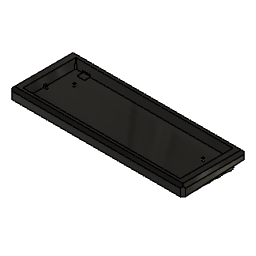
Guide_Poker (Autodesk Fusion 360 design; units mm, degrees)
Autodesk Fusion 360 part; units mm, degrees
sketch "スケッチ1" plane through (0, 0, 0) normal (0, 0, 1) x (1, 0, 0)
  line L0 (0, 0) -> (286.75, 0)
  line L1 (286.75, 0) -> (286.75, -96.25)
  line L2 (286.75, -96.25) -> (0, -96.25)
  line L3 (0, -96.25) -> (0, 0)
  line L4 (-15, 10) -> (301.75, 10)
  line L5 (301.75, 10) -> (301.75, -106.25)
  line L6 (301.75, -106.25) -> (-15, -106.25)
  line L7 (-15, -106.25) -> (-15, 10)
  circle A0 centre (260.95, -28.5) radius 2
  circle A1 centre (282.75, -57.25) radius 2
  circle A2 centre (191.45, -85.85) radius 2
  circle A3 centre (4, -57.25) radius 2
  circle A4 centre (26, -28.5) radius 2
  line L8 (286.75, -59.25) -> (282.75, -59.25)
  line L9 (286.75, -55.25) -> (282.75, -55.25)
  line L10 (0, -59.25) -> (4, -59.25)
  line L11 (0, -55.25) -> (4, -55.25)
  circle A5 centre (129, -47.75) radius 2
  circle A6 centre (4, -57.25) radius 0.9
  circle A7 centre (26, -28.5) radius 0.9
  circle A8 centre (191.45, -85.85) radius 0.9
  circle A9 centre (129, -47.75) radius 0.9
  circle A10 centre (282.75, -57.25) radius 0.9
  circle A11 centre (260.95, -28.5) radius 0.9
  dimension "d7" = 286.75
  dimension "d8" = 96.25
  dimension "d9" = 15
  dimension "d10" = 10
  dimension "d11" = 10
  dimension "d12" = 15
  dimension "d13" = 4
  dimension "d14" = 28.5
  dimension "d15" = 25.8
  dimension "d16" = 4
  dimension "d17" = 4
  dimension "d18" = 4
  dimension "d19" = 4
  dimension "d20" = 28.5
  dimension "d21" = 26
  dimension "d22" = 39
  dimension "d23" = 4
  dimension "d24" = 4
  dimension "d25" = 39
  dimension "d26" = 10.4
  dimension "d27" = 95.3
  dimension "d28" = 4
  dimension "d29" = 129
  dimension "d30" = 48.5
  dimension "d54" = 1.8
  dimension "d55" = 1.8
  dimension "d56" = 1.8
  dimension "d57" = 1.8
  dimension "d58" = 1.8
  dimension "d59" = 1.8
  constraint horizontal L0
  constraint vertical L1
  constraint horizontal L2
  constraint vertical L3
  constraint coincident L0.start L3.end
  constraint horizontal L4
  constraint vertical L5
  constraint horizontal L6
  constraint vertical L7
  constraint coincident L1 L8.start
  constraint perpendicular L1 L8
  constraint coincident L1 L9.start
  constraint perpendicular L1 L9
  constraint tangent A1 L8
  constraint tangent A1 L9
  constraint coincident A1 L8.end
  constraint coincident A1 L9.end
  constraint coincident L3 L10.start
  constraint perpendicular L3 L10
  constraint coincident L3 L11.start
  constraint perpendicular L3 L11
  constraint tangent A3 L11
  constraint tangent A3 L10
  constraint coincident A3 L10.end
  constraint coincident A3 L11.end
  constraint concentric A3 A6
  constraint concentric A4 A7
  constraint concentric A2 A8
  constraint concentric A5 A9
  constraint concentric A1 A10
  constraint concentric A0 A11
  measures "d7" distance of L1 L3
  measures "d8" distance of L0.start L2.end
  measures "d9" distance of L3 L7
  measures "d10" distance of L0 L4
  measures "d11" distance of L2 L6
  measures "d12" distance of L1 L5
  measures "d13" diameter of A0
  measures "d14" distance of L0 A0.centre
  measures "d15" distance of L1 A0.centre
  measures "d16" diameter of A1
  measures "d17" diameter of A2
  measures "d18" diameter of A3
  measures "d19" diameter of A4
  measures "d20" distance of L0 A4.centre
  measures "d21" distance of L3 A4.centre
  measures "d22" distance of L2 A3.centre
  measures "d23" distance of L3 A3.centre
  measures "d24" distance of L1 A1.centre
  measures "d25" distance of L2 A1.centre
  measures "d26" distance of L2 A2.centre
  measures "d27" distance of L1 A2.centre
  measures "d28" diameter of A5
  measures "d29" distance of L3 A5.centre
  measures "d30" distance of L2 A5.centre
  measures "d54" diameter of A6
  measures "d55" diameter of A7
  measures "d56" diameter of A8
  measures "d57" diameter of A9
  measures "d58" diameter of A10
  measures "d59" diameter of A11
extrude "押し出し1" add sketch "スケッチ1" along normal blind 14.1 contours L4 L5 L6 L7
extrude "押し出し2" add sketch "スケッチ1" against normal blind 4 contours L4 L5 L6 L7
sketch "スケッチ2" plane through (0, 0, -4) normal (0, 0, -1) x (1, 0, 0)
  line L0 (0, 96.25) -> (286.75, 96.25)
  line L1 (286.75, 96.25) -> (286.75, 0)
  line L2 (286.75, 0) -> (0, 0)
  line L3 (0, 0) -> (0, 96.25)
  line L4 (301.75, 106.25) -> (-15, 106.25)
  line L5 (-15, 106.25) -> (-15, -10)
  line L6 (-15, -10) -> (301.75, -10)
  line L7 (301.75, -10) -> (301.75, 106.25)
extrude "押し出し3" add sketch "スケッチ2" along normal blind 15 contours L0 L1 L2 L3 | L4 L5 L6 L7
sketch "スケッチ3" plane through (-15, 0, 0) normal (-1, 0, 0) x (0, -1, 0)
  line L0 (106.25, -19) -> (106.25, 14.1)
  line L1 (106.25, 14.1) -> (-10, 14.1)
  line L2 (-10, 14.1) -> (-10, -19)
  line L3 (-10, -19) -> (106.25, -19)
  line L4 (-10, -19) -> (106.25, -4.7263)
  line L5 (3.7947, -17.3062) -> (-10, 1)
  dimension "d37" = 7
  dimension "d77" = 120
  dimension "d78" = 20
  constraint coincident L2.end L3.start
  constraint coincident L0 L4.end
  constraint coincident L4 L5.start
  constraint coincident L2 L5.end
  measures "d37" angle of L3 L4
  measures "d77" angle of L4 L5
  measures "d78" distance of L2.end L5.end
extrude "押し出し4" cut sketch "スケッチ3" against normal blind 320 contours L0 L3 L4 | L2 L4 L5
extrude "押し出し5" add sketch "スケッチ1" against normal blind 4 contours L3 A3 L10 L11 | L1 A1 L8 L9 | A3 | A1 | A0 | A2 | A4 | A6 | A7 | A8 | A10 | A11
sketch "スケッチ4" plane through (0, 10, 0) normal (0, 1, 0) x (-1, 0, 0)
  line L0 (15, 1) -> (15, 14.1)
  line L1 (15, 14.1) -> (-301.75, 14.1)
  line L2 (-301.75, 14.1) -> (-301.75, 1)
  line L3 (-29, 4.6) -> (-9, 4.6)
  line L4 (-9, 4.6) -> (-9, -9.4)
  line L5 (-9, -9.4) -> (-29, -9.4)
  line L6 (-29, -9.4) -> (-29, 4.6)
  line L7 (-26, -0.4) -> (-12, -0.4)
  line L8 (-12, -0.4) -> (-12, -4.4)
  line L9 (-12, -4.4) -> (-26, -4.4)
  line L10 (-26, -4.4) -> (-26, -0.4)
  line L11 (-301.75, 1) -> (15, 1)
  dimension "d42" = 20
  dimension "d43" = 14
  dimension "d44" = 24
  dimension "d45" = 9.5
  dimension "d46" = 14
  dimension "d47" = 4
  dimension "d48" = 27
  dimension "d49" = 14.5
  constraint horizontal L3
  constraint vertical L4
  constraint horizontal L5
  constraint vertical L6
  constraint horizontal L7
  constraint vertical L8
  constraint horizontal L9
  constraint vertical L10
  measures "d42" distance of L3.start L3.end
  measures "d43" distance of L3.start L5.end
  measures "d44" distance of L0 L4
  measures "d45" distance of L1 L3
  measures "d46" distance of L7.start L7.end
  measures "d47" distance of L7.start L9.end
  measures "d48" distance of L0 L8
  measures "d49" distance of L1 L7
extrude "押し出し6" cut sketch "スケッチ4" against normal blind 20 contours L7 L8 L9 L10
extrude "押し出し7" cut sketch "スケッチ4" against normal blind 8 contours L3 L4 L6 L11 | L4 L5 L6 L11
extrude "押し出し8" cut sketch "スケッチ1" against normal blind 5 contours A6 | A7 | A8 | A10 | A11
sketch "スケッチ6" plane through (-15, 0, 0) normal (-1, 0, 0) x (0, -1, 0)
  line L0 (3.7947, -17.3062) -> (106.25, -4.7263)
  line L1 (106.25, 14.1) -> (-10, 14.1)
  line L2 (-10, 1) -> (26.6233, -14.5032)
  line L3 (-10, 1) -> (50.4444, -11.5784)
  line L4 (-10, 1) -> (106.25, -4.7263)
  line L5 (-10, 1) -> (74.2655, -8.6535)
  line L6 (-10, 1) -> (3.7947, -17.3062)
  line L7 (106.25, -4.7263) -> (106.25, 14.1)
  line L8 (-10, 14.1) -> (-10, 1)
  point P0 (-10, 1)
  dimension "d79" = 23
  dimension "d80" = 47
  dimension "d81" = 71
  dimension "d82" = 103.2247
  constraint coincident L0 L2.end
  constraint coincident L0.end L4.end
  constraint coincident L0 L5.end
  constraint coincident L0 L3.end
  constraint coincident P0 L2.start
  constraint coincident L0.start L6.end
  measures "d79" distance of L0.start L2.end
  measures "d80" distance of L0.start L3.end
  measures "d81" distance of L0.start L5.end
  measures "d82" distance of L0.start L0.end
sketch "スケッチ7" plane through (0, 10, 0) normal (0, 1, 0) x (-1, 0, 0)
  line L0 (-29, 4.6) -> (-9, 4.6)
  line L1 (-9, 1) -> (15, 1)
  line L2 (15, 14.1) -> (-301.75, 14.1)
  line L3 (15, 1) -> (10, 1)
  line L4 (10, 1) -> (10, -24)
  line L5 (10, -24) -> (15, -24)
  line L6 (15, -24) -> (15, 1)
  line L7 (10, 1) -> (7.5, 1)
  line L8 (7.5, 1) -> (7.5, -24)
  line L9 (7.5, -24) -> (10, -24)
  line L10 (10, -24) -> (10, 1)
  line L11 (7.5, 1) -> (5, 1)
  line L12 (5, 1) -> (5, -24)
  line L13 (5, -24) -> (7.5, -24)
  line L14 (7.5, -24) -> (7.5, 1)
  line L15 (5, 1) -> (2.5, 1)
  line L16 (2.5, 1) -> (2.5, -24)
  line L17 (2.5, -24) -> (5, -24)
  line L18 (5, -24) -> (5, 1)
  line L19 (15, 1) -> (15, 14.1)
  line L20 (-301.75, 14.1) -> (-301.75, 1)
  line L21 (-9, 4.6) -> (-9, 1)
  line L22 (-301.75, 1) -> (-29, 1)
  line L23 (-29, 1) -> (-29, 4.6)
  dimension "d83" = 25
  dimension "d84" = 5
  dimension "d85" = 2.5
  dimension "d86" = 25
  dimension "d87" = 2.5
  dimension "d88" = 25
  dimension "d89" = 2.5
  dimension "d90" = 25
  constraint horizontal L3
  constraint vertical L4
  constraint horizontal L5
  constraint vertical L6
  constraint horizontal L7
  constraint vertical L8
  constraint horizontal L9
  constraint vertical L10
  constraint horizontal L11
  constraint vertical L12
  constraint horizontal L13
  constraint vertical L14
  constraint horizontal L15
  constraint vertical L16
  constraint horizontal L17
  constraint vertical L18
  constraint coincident L1.end L3.start
  measures "d83" distance of L3.end L5
  measures "d84" distance of L3.end L1.end
  measures "d85" distance of L3.end L7.end
  measures "d86" distance of L3.end L4.end
  measures "d87" distance of L7.end L11.end
  measures "d88" distance of L7.end L8.end
  measures "d89" distance of L11.end L15.end
  measures "d90" distance of L11.end L12.end
sweep "スイープ1" cut profiles "スケッチ7" path "スケッチ6" along L4 section 1 contours L1 L3 L4 L5 L6 L10
sweep "スイープ2" cut profiles "スケッチ7" path "スケッチ6" along L5 section 1 contours L1 L4 L7 L8 L9 L10 L14
sweep "スイープ3" cut profiles "スケッチ7" path "スケッチ6" along L3 section 1 contours L1 L8 L11 L12 L13 L14 L18
sweep "スイープ4" cut profiles "スケッチ7" path "スケッチ6" along L2 section 1 contours L1 L12 L15 L16 L17 L18
sketch "スケッチ8" plane through (301.75, 0, 0) normal (1, 0, 0) x (0, 1, 0)
  line L0 (-106.25, -4.7263) -> (-3.7947, -17.3062)
  line L1 (-3.7947, -17.3062) -> (10, 1)
  line L2 (10, 1) -> (10, 14.1)
  line L3 (10, 14.1) -> (-106.25, 14.1)
  line L4 (-106.25, 14.1) -> (-106.25, -4.7263)
  line L5 (10, 1) -> (-106.25, -4.7263)
  line L6 (10, 1) -> (-74.2655, -8.6535)
  line L7 (10, 1) -> (-50.4444, -11.5784)
  line L8 (10, 1) -> (-26.6233, -14.5032)
  dimension "d116" = 23
  dimension "d117" = 47
  dimension "d118" = 71
  constraint coincident L1.end L2.start
  constraint coincident L0.start L4.end
  constraint coincident L0 L6.end
  constraint coincident L0 L7.end
  constraint coincident L0 L8.end
  measures "d116" distance of L0.end L8.end
  measures "d117" distance of L0.end L7.end
  measures "d118" distance of L0.end L6.end
sketch "スケッチ9" plane through (0, 10, 0) normal (0, 1, 0) x (-1, 0, 0)
  line L0 (-9, 1) -> (2.5, 1)
  line L1 (15, 1) -> (15, 14.1)
  line L2 (15, 14.1) -> (-301.75, 14.1)
  line L3 (-301.75, 14.1) -> (-301.75, 1)
  line L4 (-301.75, 1) -> (-29, 1)
  line L5 (-29, 4.6) -> (-9, 4.6)
  line L6 (-301.75, 1) -> (-296.75, 1)
  line L7 (-296.75, 1) -> (-296.75, -24)
  line L8 (-296.75, -24) -> (-301.75, -24)
  line L9 (-301.75, -24) -> (-301.75, 1)
  line L10 (-296.75, 1) -> (-294.25, 1)
  line L11 (-294.25, 1) -> (-294.25, -24)
  line L12 (-294.25, -24) -> (-296.75, -24)
  line L13 (-296.75, -24) -> (-296.75, 1)
  line L14 (-294.25, 1) -> (-291.75, 1)
  line L15 (-291.75, 1) -> (-291.75, -24)
  line L16 (-291.75, -24) -> (-294.25, -24)
  line L17 (-294.25, -24) -> (-294.25, 1)
  line L18 (-291.75, 1) -> (-289.25, 1)
  line L19 (-289.25, 1) -> (-289.25, -24)
  line L20 (-289.25, -24) -> (-291.75, -24)
  line L21 (-291.75, -24) -> (-291.75, 1)
  line L22 (-9, 4.6) -> (-9, 1)
  line L23 (2.5, 1) -> (5, 1)
  line L24 (5, 1) -> (7.5, 1)
  line L25 (7.5, 1) -> (10, 1)
  line L26 (10, 1) -> (15, 1)
  line L27 (-29, 1) -> (-29, 4.6)
  dimension "d119" = 5
  dimension "d120" = 25
  dimension "d121" = 2.5
  dimension "d122" = 25
  dimension "d123" = 2.5
  dimension "d124" = 25
  dimension "d125" = 2.5
  dimension "d126" = 25
  constraint horizontal L6
  constraint vertical L7
  constraint horizontal L8
  constraint vertical L9
  constraint coincident L3.end L4.start
  constraint horizontal L10
  constraint vertical L11
  constraint horizontal L12
  constraint vertical L13
  constraint horizontal L14
  constraint vertical L15
  constraint horizontal L16
  constraint vertical L17
  constraint horizontal L18
  constraint vertical L19
  constraint horizontal L20
  constraint vertical L21
  measures "d119" distance of L3.end L6.end
  measures "d120" distance of L3.end L8.end
  measures "d121" distance of L6.end L10.end
  measures "d122" distance of L6.end L7.end
  measures "d123" distance of L10.end L14.end
  measures "d124" distance of L10.end L11.end
  measures "d125" distance of L14.end L18.end
  measures "d126" distance of L14.end L15.end
sweep "スイープ5" cut profiles "スケッチ9" path "スケッチ8" along L5 section 1 contours L4 L6 L7 L8 L9 L13
sweep "スイープ6" cut profiles "スケッチ9" path "スケッチ8" along L6 section 1 contours L4 L7 L10 L11 L12 L13 L17
sweep "スイープ7" cut profiles "スケッチ9" path "スケッチ8" along L7 section 1 contours L4 L11 L14 L15 L16 L17 L21
sweep "スイープ8" cut profiles "スケッチ9" path "スケッチ8" along L8 section 1 contours L4 L15 L18 L19 L20 L21
fillet "フィレット6" radius 2 4 edges at (0, 0, 5.05) (0, -96.25, 5.05) (286.75, -96.25, 5.05) (286.75, 0, 5.05)
sketch "スケッチ11" plane through (0, 0, 14.1) normal (0, 0, 1) x (-1, 0, 0)
  line L0 (-284.75, 96.25) -> (-2, 96.25)
  arc A0 (0, 94.25) -> (-2, 96.25) centre (-2, 94.25) ccw
  line L1 (0, 94.25) -> (0, 2)
  arc A1 (-2, 0) -> (0, 2) centre (-2, 2) ccw
  line L2 (-2, 0) -> (-284.75, 0)
  arc A2 (-286.75, 2) -> (-284.75, 0) centre (-284.75, 2) ccw
  line L3 (-286.75, 2) -> (-286.75, 94.25)
  arc A3 (-284.75, 96.25) -> (-286.75, 94.25) centre (-284.75, 94.25) ccw
  line L4 (15, 106.25) -> (-301.75, 106.25)
  line L5 (-301.75, 106.25) -> (-301.75, -10)
  line L6 (-301.75, -10) -> (15, -10)
  line L7 (15, -10) -> (15, 106.25)
  line L8 (0, 0) -> (-286.75, 0)
  line L9 (-286.75, 0) -> (-286.75, 96.25)
  line L10 (-286.75, 96.25) -> (0, 96.25)
  line L11 (0, 96.25) -> (0, 0)
  constraint horizontal L8
  constraint vertical L9
  constraint horizontal L10
  constraint vertical L11
  constraint coincident L8.start L11.end
  constraint coincident L3.end L9
  constraint coincident L0.start L10
extrude "押し出し11" cut sketch "スケッチ11" against normal blind 9 contours A3 L9 L10 | A0 L10 L11 | A2 L8 L9 | A1 L8 L11
fillet "フィレット7" radius 1 4 edges at (286.75, 0, 9.6) (286.75, -96.25, 9.6) (0, -96.25, 9.6) (0, 0, 9.6)
fillet "フィレット5" radius 5 4 edges at (9, 6, 4.6) (9, 2.0815, -9.4) (29, 2.0815, -9.4) (29, 6, 4.6)
chamfer "面取り2" distance 5 angle 45 4 edges at (301.75, -106.25, 4.6869) (301.75, 10, 7.55) (-15, 10, 7.55) (-15, -106.25, 4.6869)
chamfer "面取り3" distance 5 angle 45 4 edges at (301.75, -48.125, 14.1) (143.375, -106.25, 14.1) (143.375, 10, 14.1) (-15, -48.125, 14.1)
chamfer "面取り6" distance 0.5 angle 45 1 edges at (301.75, -48.125, -1.8631)
chamfer "面取り6" distance 0.1 angle 45 7 edges at (9, 7.4379, -2.4) (9.0503, 9.4779, 0.3071) (28.9497, 9.4779, 0.3071) (29, 7.4379, -2.4) (27.5355, 3.2666, -7.9355) (19, 2.163, -9.4) (10.4645, 3.2666, -7.9355)
chamfer "面取り6" distance 1 angle 45 3 edges at (11, 10, 3.6) (27, 10, 3.6) (19, 10, 4.6)
chamfer "面取り7" distance 0.5 angle 45 2 edges at (143.375, -3.7947, -17.3062) (143.375, -106.25, -4.7263)
equation "d7 = ( 19.05 * 15 ) * 1 mm + ( 0.5 * 2 ) * 1 mm"
equation "d8 = ( 19.05 * 5 ) * 1 mm + ( 0.5 * 2 ) * 1 mm"
equation "d14 = 28 mm + 0.5 mm"
equation "d15 = 25.3 mm + 0.5 mm"
equation "d20 = 28 mm + 0.5 mm"
equation "d21 = 25.5 mm + 0.5 mm"
equation "d22 = 38.5 mm + 0.5 mm"
equation "d23 = 3.5 mm + 0.5 mm"
equation "d24 = 3.5 mm + 0.5 mm"
equation "d25 = 38.5 mm + 0.5 mm"
equation "d26 = 9.9 mm + 0.5 mm"
equation "d27 = 94.8 mm + 0.5 mm"
equation "d29 = 128.5 mm + 0.5 mm"
equation "d30 = 48 mm + 0.5 mm"
equation "d31 = 7.5 mm + 5 mm + 1.6 mm"
equation "d33 = -2 mm - 2 mm"
equation "d44 = 9 mm + 15 mm"
equation "d48 = 12 mm + 15 mm"
equation "d80 = ( 23 * 2 ) * 1 mm + 1 mm"
equation "d81 = ( 23 * 3 ) * 1 mm + 2 mm"
equation "d117 = ( 23 * 2 ) * 1 mm + 1 mm"
equation "d118 = ( 23 * 3 ) * 1 mm + 2 mm"
